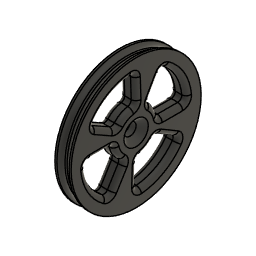
4c26e493-739a-48ea-874f-1be753068770 (Autodesk Fusion 360 design; units mm, degrees)
Autodesk Fusion 360 part; units mm, degrees
sketch "Esboço3" plane through (0, 0, 0) normal (1, 0, 0) x (0, 1, 0)
  circle A0 centre (82.9895, -0.0021) radius 16
  circle A1 centre (82.9895, -0.0021) radius 3.25
  circle A2 centre (82.9895, -0.0021) radius 1.5
  line L0 (86.3652, 5.4051) -> (88.8333, 9.8205)
  line L1 (89.3865, 0.1504) -> (94.4316, 0.1504)
  line L2 (82.977, 6.4515) -> (82.8119, 11.4704)
  line L3 (77.5688, 3.3637) -> (73.1661, 5.847)
  line L4 (76.5935, -0.1579) -> (71.5479, -0.1559)
  line L5 (79.7376, -5.5624) -> (77.1193, -9.8526)
  line L6 (83.251, -6.3492) -> (83.1018, -11.4189)
  line L7 (88.4797, -3.3172) -> (92.8163, -5.8815)
  arc A3 (88.4024, 0.9731) -> (86.5845, 4.1603) centre (82.9895, -0.0021) ccw
  arc A4 (95.4266, 1.2507) -> (90.2903, 10.1442) centre (82.9895, -0.0021) ccw
  arc A5 (84.1981, -12.4436) -> (93.1175, -7.3284) centre (82.9895, -0.0021) ccw
  arc A6 (84.0565, -5.3976) -> (87.2044, -3.5356) centre (82.9895, -0.0021) ccw
  arc A7 (81.7101, 12.4322) -> (72.8458, 7.3024) centre (82.9895, -0.0021) ccw
  arc A8 (70.5526, -1.2563) -> (75.6811, -10.143) centre (82.9895, -0.0021) ccw
  arc A9 (82.1333, 5.4308) -> (78.8185, 3.5829) centre (82.9895, -0.0021) ccw
  arc A10 (77.5772, -0.9801) -> (79.5156, -4.2662) centre (82.9895, -0.0021) ccw
  arc A11 (82.8119, 11.4704) -> (81.7101, 12.4322) centre (81.8124, 11.4375) ccw
  arc A12 (82.1333, 5.4308) -> (82.977, 6.4515) centre (81.9776, 6.4186) ccw
  arc A13 (77.5688, 3.3637) -> (78.8185, 3.5829) centre (78.0601, 4.2347) ccw
  arc A14 (72.8458, 7.3024) -> (73.1661, 5.847) centre (73.6573, 6.718) ccw
  arc A15 (71.5479, -0.1559) -> (70.5526, -1.2563) centre (71.5476, -1.1559) ccw
  arc A16 (77.5772, -0.9801) -> (76.5935, -0.1579) centre (76.5931, -1.1579) ccw
  arc A17 (79.7376, -5.5624) -> (79.5156, -4.2662) centre (78.884, -5.0415) ccw
  arc A18 (75.6811, -10.143) -> (77.1193, -9.8526) centre (76.2657, -9.3317) ccw
  arc A19 (84.0565, -5.3976) -> (83.251, -6.3492) centre (84.2505, -6.3786) ccw
  arc A20 (88.4797, -3.3172) -> (87.2044, -3.5356) centre (87.9707, -4.178) ccw
  arc A21 (93.1175, -7.3284) -> (92.8163, -5.8815) centre (92.3073, -6.7423) ccw
  arc A22 (83.1018, -11.4189) -> (84.1981, -12.4436) centre (84.1014, -11.4483) ccw
  arc A23 (94.4316, 0.1504) -> (95.4266, 1.2507) centre (94.4316, 1.1504) ccw
  arc A24 (90.2903, 10.1442) -> (88.8333, 9.8205) centre (89.7062, 9.3325) ccw
  arc A25 (86.3652, 5.4051) -> (86.5845, 4.1603) centre (87.2381, 4.9172) ccw
  arc A26 (88.4024, 0.9731) -> (89.3865, 0.1504) centre (89.3865, 1.1504) ccw
  line L8 (85.8395, 2.8479) -> (80.1395, -2.8521) construction
  line L9 (80.1395, 2.8479) -> (85.8395, -2.8521) construction
  circle A27 centre (82.9895, -0.0021) radius 15.25
  point P0 (82.9895, -0.0021)
  dimension "d388_2_1" = 32
  dimension "d389_2_1" = 6.5
  dimension "d390_2_1" = 3
  dimension "d391_2_1" = 11
  dimension "d392_2_1" = 25
  dimension "d393_2_1" = 1
  dimension "d431_1" = 30.5
  constraint concentric A0 A7
  constraint concentric A7 A9
  constraint concentric A1 A9
  constraint concentric A1 A2
  constraint horizontal L1
  constraint concentric A3 A9
  constraint concentric A4 A7
  constraint concentric A5 A7
  constraint concentric A6 A9
  constraint concentric A7 A8
  constraint concentric A9 A10
  constraint tangent A7 A11
  constraint tangent L2 A11
  constraint tangent L2 A12
  constraint tangent A9 A12
  constraint equal A11 A12
  constraint tangent A9 A13
  constraint tangent L3 A13
  constraint equal A11 A13
  constraint tangent L3 A14
  constraint tangent A7 A14
  constraint equal A11 A14
  constraint tangent L4 A15
  constraint tangent A8 A15
  constraint equal A11 A15
  constraint tangent L4 A16
  constraint tangent A10 A16
  constraint equal A11 A16
  constraint tangent A10 A17
  constraint tangent L5 A17
  constraint equal A11 A17
  constraint tangent L5 A18
  constraint tangent A8 A18
  constraint equal A11 A18
  constraint tangent L6 A19
  constraint tangent A6 A19
  constraint equal A11 A19
  constraint tangent A6 A20
  constraint tangent L7 A20
  constraint equal A11 A20
  constraint tangent L7 A21
  constraint tangent A5 A21
  constraint equal A11 A21
  constraint tangent A5 A22
  constraint tangent L6 A22
  constraint equal A11 A22
  constraint tangent L1 A23
  constraint tangent A4 A23
  constraint equal A11 A23
  constraint tangent A4 A24
  constraint tangent L0 A24
  constraint equal A11 A24
  constraint tangent L0 A25
  constraint tangent A3 A25
  constraint equal A11 A25
  constraint tangent A3 A26
  constraint tangent L1 A26
  constraint equal A11 A26
  constraint coincident L8 P0
  constraint coincident L9 P0
  constraint coincident P0 A0.centre
  constraint equal A4 A7
  constraint equal A5 A7
  constraint equal A7 A8
  constraint concentric A9 A27
  constraint equal A3 A9
  constraint equal A6 A9
  constraint equal A9 A10
  measures "d388_2_1" diameter of A0
  measures "d389_2_1" diameter of A1
  measures "d390_2_1" diameter of A2
  measures "d391_2_1" diameter of A9
  measures "d392_2_1" diameter of A7
  measures "d393_2_1" radius of A11
  measures "d431_1" diameter of A27
extrude "Extrusão1" add sketch "Esboço3" along normal blind 4 contours A0 | A1 | A27
extrude "Extrusão2" cut sketch "Esboço3" along normal blind 1 contours A1
fillet "Arredondamento1" radius 1.2 64 edges at (4, 75.3674, 4.6053) (4, 72.6807, 6.5031) (4, 76.7285, 10.8168) (4, 82.47, 12.1908) (4, 82.8944, 8.9609) (4, 82.7483, 5.7815) (4, 80.3114, 4.8018) (4, 78.2328, 3.2497) (4, 87.5993, 7.6128) (4, 89.4893, 10.3087) (4, 93.814, 6.2493) (4, 95.1733, 0.4797) (4, 91.9091, 0.1504) (4, 88.7452, 0.3832) (4, 87.767, 2.7228) (4, 86.2533, 4.7437) (4, 78.4285, -7.7075) (4, 76.4636, -10.3119) (4, 72.163, -6.2501) (4, 70.8059, -0.4851) (4, 74.0707, -0.1569) (4, 77.2344, -0.3906) (4, 78.2523, -2.7966) (4, 79.8697, -4.8727) (4, 90.648, -4.5994) (4, 93.2863, -6.5384) (4, 89.2081, -10.8455) (4, 83.4185, -12.1788) (4, 83.1764, -8.884) (4, 83.4873, -5.7325) (4, 85.7898, -4.7359) (4, 87.802, -3.1923) (0, 90.648, -4.5994) (0, 93.2863, -6.5384) (0, 89.2081, -10.8455) (0, 83.4185, -12.1788) (0, 83.1764, -8.884) (0, 83.4873, -5.7325) (0, 85.7898, -4.7359) (0, 87.802, -3.1923) (0, 72.163, -6.2501) (0, 70.8059, -0.4851) (0, 74.0707, -0.1569) (0, 77.2344, -0.3906) (0, 78.2523, -2.7966) (0, 79.8697, -4.8727) (0, 78.4285, -7.7075) (0, 76.4636, -10.3119) (0, 87.5993, 7.6128) (0, 89.4893, 10.3087) (0, 93.814, 6.2493) (0, 95.1733, 0.4797) (0, 91.9091, 0.1504) (0, 88.7452, 0.3832) (0, 87.767, 2.7228) (0, 86.2533, 4.7437) (0, 80.3114, 4.8018) (0, 78.2328, 3.2497) (0, 75.3674, 4.6053) (0, 72.6807, 6.5031) (0, 76.7285, 10.8168) (0, 82.47, 12.1908) (0, 82.8944, 8.9609) (0, 82.7483, 5.7815)
chamfer "Chanfro1" distance 1.5 angle 45 1 edges at (4, 81.591, 0.5403)
extrude "Extrusão3" cut sketch "Esboço3" along normal blind 0.5 and the other way blind -3.5 contours A0
fillet "Arredondamento2" radius 1.4 2 edges at (3.5, 68.7715, 5.5125) (0.5, 68.7715, 5.5125)
